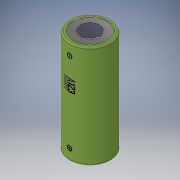
# Autodesk Inventor part: Battery Cell
Saved by Autodesk Inventor 2019.2 (Build 232265000, 265)
## iProperties
Created: 2018-12-05
Part Number: Battery Cell
Material: Nickel-Copper Alloy 400
Document SubType Name: Modeling
Designer: Petar
Density: 8.83 g/cm^3
Appearance: Chrome - Polished
Author: Petar
Autodesk Inventor part; units mm, degrees
ref_plane "YZ Plane" through (0, 0, 0) normal (1, 0, 0) x (0, 1, 0)
ref_plane "XZ Plane" through (0, 0, 0) normal (0, 1, 0) x (-1, 0, 0)
sketch "Sketch1" plane through (0, 0, 0) normal (1, 0, 0) x (0, 1, 0)
  line L0 (0, 0) -> (65, 0)
  line L1 (65, 0) -> (65, 13)
  line L2 (65, 13) -> (0, 13)
  line L3 (0, 13) -> (0, 0)
  dimension "d0" = 65
  dimension "d1" = 13
  constraints: 8 end point, 2 perpendicular, 1 horizontal, 1 vertical
  measures "d0" distance of L0.start L0.end
  measures "d1" distance of L0.end L1.end
revolve "Revolution1" add sketch "Sketch1" angle 360 about axis through (0, 0, 0) along (0, 1, 0)
fillet "Fillet1" radius 1 2 edges at (0, 65, -13) (0, 0, -13)
sketch "Sketch2" plane through (0, 65, 0) normal (0, 1, 0) x (1, 0, 0)
  circle A0 centre (0, 0) radius 12 projected
  circle A1 centre (0, 0) radius 6.5
  circle A2 centre (0, 0) radius 10.5
  dimension "d4" = 13
  dimension "d5" = 21
  constraints: 2 centre point, 2 coincident
  measures "d4" diameter of A1
  measures "d5" diameter of A2
extrude "Extrusion1" cut sketch "Sketch2" against normal blind 0.2 contours A2
fillet "Fillet2" radius 0.5 2 edges at (-10.5, 65, 0) (-6.5, 65, 0)
sketch "Sketch5" plane through (0, 0, 0) normal (0, -1, 0) x (1, 0, 0)
  circle A0 centre (0, 0) radius 10.9 projected
extrude "Extrusion2" cut sketch "Sketch5" against normal blind 0.2
ref_plane "Work Plane1" through (0, 65, 13) normal (0, 0, 1) x (1, 0, 0)
sketch "Sketch3" plane through (0, 65, 13) normal (0, 0, 1) x (1, 0, 0)
  line L0 (1.2249, -5) -> (1.2249, -9.446) construction
  line L1 (1.2249, -9.446) -> (-1.2249, -9.446) construction
  line L2 (-1.2249, -9.446) -> (-1.2249, -5) construction
  line L3 (-1.2249, -5) -> (1.2249, -5) construction
  line L4 (0, -65) -> (0, -0.9999) construction
  line L5 (1.8449, -55.554) -> (1.8449, -60) construction
  line L6 (1.8449, -60) -> (-1.8449, -60) construction
  line L7 (-1.8449, -60) -> (-1.8449, -55.554) construction
  line L8 (-1.8449, -55.554) -> (1.8449, -55.554) construction
  line L9 (-4.7875, -3) -> (4.7875, -3) construction
  line L10 (4.7875, -3) -> (4.7875, -11.446) construction
  line L11 (4.7875, -11.446) -> (-4.7875, -11.446) construction
  line L12 (-4.7875, -11.446) -> (-4.7875, -3) construction
  line L13 (-4.7783, -53.554) -> (4.7783, -53.554) construction
  line L14 (4.7783, -53.554) -> (4.7783, -62) construction
  line L15 (4.7783, -62) -> (-4.7783, -62) construction
  line L16 (-4.7783, -62) -> (-4.7783, -53.554) construction
  line L17 (13, -1) -> (-13, -1) construction
  line L18 (-13, -64) -> (13, -64) construction
  spline S0 degree 2 poles (1.1765, -6.0465) (1.3866, -6.2492) (1.6165, -6.8424) (1.6165, -7.223) knots 0 0 0 1 2 2 2
  spline S1 degree 2 poles (1.6165, -7.223) (1.6165, -7.5937) (1.3915, -8.1943) (1.1765, -8.397) knots 0 0 0 1 2 2 2
  spline S2 degree 2 poles (1.1765, -8.397) (0.9541, -8.6096) (0.3584, -8.8123) (0, -8.8123) knots 0 0 0 1 2 2 2
  spline S3 degree 2 poles (0, -8.8123) (-0.3707, -8.8123) (-0.9664, -8.6022) (-1.179, -8.397) knots 0 0 0 1 2 2 2
  spline S4 degree 2 poles (-1.179, -8.397) (-1.3915, -8.1943) (-1.6165, -7.5987) (-1.6165, -7.223) knots 0 0 0 1 2 2 2
  spline S5 degree 2 poles (-1.6165, -7.223) (-1.6165, -6.8399) (-1.3891, -6.2566) (-1.1765, -6.0465) knots 0 0 0 1 2 2 2
  spline S6 degree 2 poles (-1.1765, -6.0465) (-0.9664, -5.8438) (-0.3683, -5.6337) (0, -5.6337) knots 0 0 0 1 2 2 2
  spline S7 degree 2 poles (0, -5.6337) (0.3707, -5.6337) (0.9714, -5.8512) (1.1765, -6.0465) knots 0 0 0 1 2 2 2
  spline S8 degree 2 poles (1.1098, -7.223) (1.1098, -6.9214) (0.9541, -6.4543) (0.8107, -6.3011) knots 0 0 0 1 2 2 2
  spline S9 degree 2 poles (0.8107, -6.3011) (0.6649, -6.1429) (0.2571, -5.9847) (0.0025, -5.9847) knots 0 0 0 1 2 2 2
  spline S10 degree 2 poles (0.0025, -5.9847) (-0.2645, -5.9847) (-0.6575, -6.1379) (-0.8107, -6.3011) knots 0 0 0 1 2 2 2
  spline S11 degree 2 poles (-0.8107, -6.3011) (-0.9541, -6.4568) (-1.1098, -6.9264) (-1.1098, -7.223) knots 0 0 0 1 2 2 2
  spline S12 degree 2 poles (-1.1098, -7.223) (-1.1098, -7.8236) (-0.5067, -8.4613) (0.0025, -8.4613) knots 0 0 0 1 2 2 2
  spline S13 degree 2 poles (0.0025, -8.4613) (0.5092, -8.4613) (1.1098, -7.8236) (1.1098, -7.223) knots 0 0 0 1 2 2 2
  line L19 (-0.1957, -6.3278) -> (0.1957, -6.3278)
  line L20 (0.1957, -6.3278) -> (0.1957, -8.1206)
  line L21 (0.1957, -8.1206) -> (-0.1957, -8.1206)
  line L22 (-0.1957, -8.1206) -> (-0.1957, -6.3278)
  spline S14 degree 2 poles (1.1765, -56.6005) (1.3866, -56.8032) (1.6165, -57.3964) (1.6165, -57.777) knots 0 0 0 1 2 2 2
  spline S15 degree 2 poles (1.6165, -57.777) (1.6165, -58.1478) (1.3915, -58.7484) (1.1765, -58.951) knots 0 0 0 1 2 2 2
  spline S16 degree 2 poles (1.1765, -58.951) (0.9541, -59.1636) (0.3584, -59.3663) (0, -59.3663) knots 0 0 0 1 2 2 2
  spline S17 degree 2 poles (0, -59.3663) (-0.3707, -59.3663) (-0.9664, -59.1562) (-1.179, -58.951) knots 0 0 0 1 2 2 2
  spline S18 degree 2 poles (-1.179, -58.951) (-1.3915, -58.7484) (-1.6165, -58.1527) (-1.6165, -57.777) knots 0 0 0 1 2 2 2
  spline S19 degree 2 poles (-1.6165, -57.777) (-1.6165, -57.3939) (-1.3891, -56.8106) (-1.1765, -56.6005) knots 0 0 0 1 2 2 2
  spline S20 degree 2 poles (-1.1765, -56.6005) (-0.9664, -56.3978) (-0.3683, -56.1877) (0, -56.1877) knots 0 0 0 1 2 2 2
  spline S21 degree 2 poles (0, -56.1877) (0.3707, -56.1877) (0.9714, -56.4053) (1.1765, -56.6005) knots 0 0 0 1 2 2 2
  spline S22 degree 2 poles (1.1098, -57.777) (1.1098, -57.4755) (0.9541, -57.0083) (0.8107, -56.8551) knots 0 0 0 1 2 2 2
  spline S23 degree 2 poles (0.8107, -56.8551) (0.6649, -56.6969) (0.2571, -56.5387) (0.0025, -56.5387) knots 0 0 0 1 2 2 2
  spline S24 degree 2 poles (0.0025, -56.5387) (-0.2645, -56.5387) (-0.6575, -56.692) (-0.8107, -56.8551) knots 0 0 0 1 2 2 2
  spline S25 degree 2 poles (-0.8107, -56.8551) (-0.9541, -57.0108) (-1.1098, -57.4804) (-1.1098, -57.777) knots 0 0 0 1 2 2 2
  spline S26 degree 2 poles (-1.1098, -57.777) (-1.1098, -58.3776) (-0.5067, -59.0153) (0.0025, -59.0153) knots 0 0 0 1 2 2 2
  spline S27 degree 2 poles (0.0025, -59.0153) (0.5092, -59.0153) (1.1098, -58.3776) (1.1098, -57.777) knots 0 0 0 1 2 2 2
  line L23 (-1.0474, -57.5934) -> (-0.1776, -57.5934)
  line L24 (-0.1776, -57.5934) -> (-0.1776, -56.7308)
  line L25 (-0.1776, -56.7308) -> (0.1848, -56.7308)
  line L26 (0.1848, -56.7308) -> (0.1848, -57.5934)
  line L27 (0.1848, -57.5934) -> (1.0474, -57.5934)
  line L28 (1.0474, -57.5934) -> (1.0474, -57.9606)
  line L29 (1.0474, -57.9606) -> (0.1848, -57.9606)
  line L30 (0.1848, -57.9606) -> (0.1848, -58.8232)
  line L31 (0.1848, -58.8232) -> (-0.1776, -58.8232)
  line L32 (-0.1776, -58.8232) -> (-0.1776, -57.9606)
  line L33 (-0.1776, -57.9606) -> (-1.0474, -57.9606)
  line L34 (-1.0474, -57.9606) -> (-1.0474, -57.5934)
  dimension "d9" = 2
  dimension "d10" = 2
  dimension "d11" = 2
  dimension "d12" = 2
  dimension "d13" = 2
  dimension "d14" = 2
  constraints: 2 end point, 1 vertical, 12 other
  measures "d9" distance between parallel lines of L11 L1
  measures "d10" distance between parallel lines of L9 L3
  measures "d11" distance between parallel lines of L8 L13
  measures "d12" distance between parallel lines of L15 L6
  measures "d13" distance between parallel lines of L9 L17
  measures "d14" distance between parallel lines of L18 L15
emboss "Emboss1" sketch "Sketch3" operation cut depth 0.01 direction (0, 0, -1) draft 1
sketch "Sketch4" plane through (0, 65, 13) normal (0, 0, 1) x (1, 0, 0)
  line L0 (-6.1, 0) -> (6.1, 0) construction
  line L1 (0, 0) -> (0, -65) construction
  line L2 (3.5, -19) -> (3.5, -28) construction
  line L3 (3.5, -28) -> (-0.8355, -28) construction
  line L4 (-0.8355, -28) -> (-0.8355, -19) construction
  line L5 (-0.8355, -19) -> (3.5, -19) construction
  line L6 (-0.9355, -19) -> (-0.9355, -28) construction
  line L7 (-0.9355, -28) -> (-4.5, -28) construction
  line L8 (-4.5, -28) -> (-4.5, -19) construction
  line L9 (-4.5, -19) -> (-0.9355, -19) construction
  line L10 (3.2329, -20.5357) -> (-0.7671, -21.3601)
  line L11 (-0.7671, -21.3601) -> (-0.7671, -20.7321)
  line L12 (-0.7671, -20.7321) -> (-0.2046, -20.625)
  line L13 (-0.2046, -20.625) -> (-0.2046, -19.8363)
  line L14 (-0.2046, -19.8363) -> (-0.7671, -19.7351)
  line L15 (-0.7671, -19.7351) -> (-0.7671, -19.1071)
  line L16 (-0.7671, -19.1071) -> (3.2329, -19.9077)
  line L17 (3.2329, -19.9077) -> (3.2329, -20.5357)
  line L18 (0.2805, -19.9196) -> (0.2805, -20.5446)
  line L19 (0.2805, -20.5446) -> (2.1317, -20.2262)
  line L20 (2.1317, -20.2262) -> (0.2805, -19.9196)
  spline S0 degree 2 poles (2.9085, -21.7827) (2.9085, -21.9048) (3.0484, -22.006) (3.2329, -22.006) knots 0 0 0 1 2 2 2
  line L21 (3.2329, -22.006) -> (3.2329, -22.6607)
  line L22 (3.2329, -22.6607) -> (-0.7671, -22.6607)
  line L23 (-0.7671, -22.6607) -> (-0.7671, -22.006)
  line L24 (-0.7671, -22.006) -> (2.4234, -22.006)
  line L25 (2.4234, -22.006) -> (2.4234, -21.503)
  line L26 (2.4234, -21.503) -> (2.9085, -21.503)
  line L27 (2.9085, -21.503) -> (2.9085, -21.7827)
  spline S1 degree 2 poles (3.3014, -24.0208) (3.3014, -24.4583) (2.8668, -25.003) (2.3906, -25.003) knots 0 0 0 1 2 2 2
  spline S2 degree 2 poles (2.3906, -25.003) (2.1734, -25.003) (1.8639, -24.8839) (1.7002, -24.7738) knots 0 0 0 1 2 2 2
  spline S3 degree 2 poles (1.7002, -24.7738) (1.599, -24.7024) (1.3103, -24.4554) (1.0305, -24.2083) (0.7865, -24.0327) (0.6406, -23.9107) knots 0 0 0 1 2 3 4 4 4
  spline S4 degree 2 poles (0.6406, -23.9107) (0.5811, -23.878) (0.4353, -23.7946) (0.3073, -23.75) (0.1615, -23.7321) (0.0514, -23.7321) knots 0 0 0 1 2 3 4 4 4
  line L28 (0.0514, -23.7321) -> (-0.2225, -23.7321)
  line L29 (-0.2225, -23.7321) -> (-0.2225, -25.003)
  line L30 (-0.2225, -25.003) -> (-0.7671, -25.003)
  line L31 (-0.7671, -25.003) -> (-0.7671, -23.0774)
  line L32 (-0.7671, -23.0774) -> (0.0514, -23.0774)
  spline S5 degree 2 poles (0.0514, -23.0774) (0.2478, -23.0774) (0.6347, -23.1845) (0.8549, -23.3333) knots 0 0 0 1 2 2 2
  spline S6 degree 2 poles (0.8549, -23.3333) (0.9531, -23.4018) (1.227, -23.631) (1.5127, -23.875) (1.7805, -24.1071) (1.8906, -24.1815) knots 0 0 0 1 2 3 4 4 4
  spline S7 degree 2 poles (1.8906, -24.1815) (2.0335, -24.2798) (2.2805, -24.3542) (2.4055, -24.3542) knots 0 0 0 1 2 2 2
  spline S8 degree 2 poles (2.4055, -24.3542) (2.6049, -24.3542) (2.7567, -24.1786) (2.7567, -24.0089) knots 0 0 0 1 2 2 2
  spline S9 degree 2 poles (2.7567, -24.0089) (2.7567, -23.8304) (2.6168, -23.6488) (2.471, -23.6488) knots 0 0 0 1 2 2 2
  line L33 (2.471, -23.6488) -> (2.3014, -23.6488)
  line L34 (2.3014, -23.6488) -> (2.3014, -23.0357)
  line L35 (2.3014, -23.0357) -> (2.4799, -23.0357)
  spline S10 degree 2 poles (2.4799, -23.0357) (2.8609, -23.0357) (3.3014, -23.5536) (3.3014, -24.0208) knots 0 0 0 1 2 2 2
  spline S11 degree 2 poles (3.3014, -26.2411) (3.3014, -26.4851) (3.1674, -26.8542) (2.9264, -27.1131) (2.596, -27.2411) (2.4115, -27.2411) knots 0 0 0 1 2 3 4 4 4
  line L36 (2.4115, -27.2411) -> (1.8668, -27.2411)
  spline S12 degree 2 poles (1.8668, -27.2411) (1.6139, -27.2411) (1.3222, -27.0565) (1.3073, -26.8988) knots 0 0 0 1 2 2 2
  spline S13 degree 2 poles (1.3073, -26.8988) (1.2895, -27.0685) (0.9799, -27.2946) (0.7061, -27.2946) knots 0 0 0 1 2 2 2
  line L37 (0.7061, -27.2946) -> (-0.0201, -27.2946)
  spline S14 degree 2 poles (-0.0201, -27.2946) (-0.2105, -27.2946) (-0.5171, -27.1339) (-0.7284, -26.8542) (-0.8355, -26.4851) (-0.8355, -26.2708) knots 0 0 0 1 2 3 4 4 4
  spline S15 degree 2 poles (-0.8355, -26.2708) (-0.8355, -26.0565) (-0.7284, -25.6964) (-0.5111, -25.4286) (-0.2046, -25.2798) (-0.0141, -25.2798) knots 0 0 0 1 2 3 4 4 4
  line L38 (-0.0141, -25.2798) -> (0.2359, -25.2798)
  line L39 (0.2359, -25.2798) -> (0.1139, -25.8929)
  line L40 (0.1139, -25.8929) -> (-0.0052, -25.8929)
  spline S16 degree 2 poles (-0.0052, -25.8929) (-0.151, -25.8929) (-0.2939, -26.0893) (-0.2939, -26.2649) knots 0 0 0 1 2 2 2
  spline S17 degree 2 poles (-0.2939, -26.2649) (-0.2939, -26.4464) (-0.148, -26.6458) (-0.0052, -26.6458) knots 0 0 0 1 2 2 2
  line L41 (-0.0052, -26.6458) -> (0.7121, -26.6458)
  spline S18 degree 2 poles (0.7121, -26.6458) (0.8996, -26.6458) (1.0454, -26.4851) (1.0454, -26.2649) knots 0 0 0 1 2 2 2
  line L42 (1.0454, -26.2649) -> (1.0454, -25.8839)
  line L43 (1.0454, -25.8839) -> (1.5395, -25.8839)
  line L44 (1.5395, -25.8839) -> (1.5395, -26.2292)
  spline S19 degree 2 poles (1.5395, -26.2292) (1.5395, -26.4375) (1.6734, -26.5982) (1.852, -26.5982) knots 0 0 0 1 2 2 2
  line L45 (1.852, -26.5982) -> (2.4145, -26.5982)
  spline S20 degree 2 poles (2.4145, -26.5982) (2.5781, -26.5982) (2.7567, -26.4345) (2.7567, -26.2351) knots 0 0 0 1 2 2 2
  spline S21 degree 2 poles (2.7567, -26.2351) (2.7567, -26.0536) (2.6049, -25.8929) (2.4502, -25.8929) knots 0 0 0 1 2 2 2
  line L46 (2.4502, -25.8929) -> (2.3014, -25.8929)
  line L47 (2.3014, -25.8929) -> (2.3014, -25.2798)
  line L48 (2.3014, -25.2798) -> (2.4799, -25.2798)
  spline S22 degree 2 poles (2.4799, -25.2798) (2.8609, -25.2798) (3.3014, -25.8036) (3.3014, -26.2411) knots 0 0 0 1 2 2 2
  line L49 (-1.7706, -19.075) -> (-1.7578, -19.225)
  spline S23 degree 2 poles (-1.7578, -19.225) (-1.8484, -19.236) (-1.9636, -19.3137) (-2.0349, -19.4774) (-2.0349, -19.5799) knots 0 0 0 1 2 3 3 3
  spline S24 degree 2 poles (-2.0349, -19.5799) (-2.0349, -19.6704) (-1.981, -19.8104) (-1.8868, -19.878) (-1.831, -19.878) knots 0 0 0 1 2 3 3 3
  spline S25 degree 2 poles (-1.831, -19.878) (-1.7743, -19.878) (-1.6901, -19.8131) (-1.6618, -19.7372) knots 0 0 0 1 2 2 2
  spline S26 degree 2 poles (-1.6618, -19.7372) (-1.6426, -19.6887) (-1.563, -19.3567) (-1.5273, -19.2899) knots 0 0 0 1 2 2 2
  spline S27 degree 2 poles (-1.5273, -19.2899) (-1.4825, -19.204) (-1.349, -19.1198) (-1.2666, -19.1198) knots 0 0 0 1 2 2 2
  spline S28 degree 2 poles (-1.2666, -19.1198) (-1.1752, -19.1198) (-1.0179, -19.2232) (-0.9355, -19.4216) (-0.9355, -19.5433) knots 0 0 0 1 2 3 3 3
  spline S29 degree 2 poles (-0.9355, -19.5433) (-0.9355, -19.6768) (-1.0215, -19.8808) (-1.1889, -19.9915) (-1.2941, -19.9951) knots 0 0 0 1 2 3 3 3
  line L50 (-1.2941, -19.9951) -> (-1.306, -19.8433)
  spline S30 degree 2 poles (-1.306, -19.8433) (-1.1916, -19.8314) (-1.0755, -19.6887) (-1.0755, -19.5497) knots 0 0 0 1 2 2 2
  spline S31 degree 2 poles (-1.0755, -19.5497) (-1.0755, -19.4052) (-1.1816, -19.2726) (-1.2557, -19.2726) knots 0 0 0 1 2 2 2
  spline S32 degree 2 poles (-1.2557, -19.2726) (-1.3206, -19.2726) (-1.3627, -19.3192) knots 0 0 0 1 1 1
  spline S33 degree 2 poles (-1.3627, -19.3192) (-1.4038, -19.3659) (-1.4916, -19.7546) (-1.5246, -19.8268) knots 0 0 0 1 2 2 2
  spline S34 degree 2 poles (-1.5246, -19.8268) (-1.573, -19.9311) (-1.7212, -20.0308) (-1.8173, -20.0308) knots 0 0 0 1 2 2 2
  spline S35 degree 2 poles (-1.8173, -20.0308) (-1.9133, -20.0308) (-2.0825, -19.921) (-2.1767, -19.7152) (-2.1767, -19.5872) knots 0 0 0 1 2 3 3 3
  spline S36 degree 2 poles (-2.1767, -19.5872) (-2.1767, -19.4235) (-2.0816, -19.204) (-1.8913, -19.0787) (-1.7706, -19.075) knots 0 0 0 1 2 3 3 3
  line L51 (-2.1566, -20.586) -> (-1.648, -20.586)
  line L52 (-1.648, -20.586) -> (-0.9566, -20.1232)
  line L53 (-0.9566, -20.1232) -> (-0.9566, -20.3162)
  line L54 (-0.9566, -20.3162) -> (-1.3188, -20.553)
  spline S37 degree 2 poles (-1.3188, -20.553) (-1.4194, -20.6198) (-1.5218, -20.6756) knots 0 0 0 1 1 1
  spline S38 degree 2 poles (-1.5218, -20.6756) (-1.4276, -20.7296) (-1.3096, -20.8064) knots 0 0 0 1 1 1
  line L55 (-1.3096, -20.8064) -> (-0.9566, -21.0396)
  line L56 (-0.9566, -21.0396) -> (-0.9566, -21.2244)
  line L57 (-0.9566, -21.2244) -> (-1.648, -20.7451)
  line L58 (-1.648, -20.7451) -> (-2.1566, -20.7451)
  line L59 (-2.1566, -20.7451) -> (-2.1566, -20.586)
  line L60 (-1.7706, -21.3122) -> (-1.7578, -21.4622)
  spline S39 degree 2 poles (-1.7578, -21.4622) (-1.8484, -21.4732) (-1.9636, -21.5509) (-2.0349, -21.7146) (-2.0349, -21.8171) knots 0 0 0 1 2 3 3 3
  spline S40 degree 2 poles (-2.0349, -21.8171) (-2.0349, -21.9076) (-1.981, -22.0476) (-1.8868, -22.1152) (-1.831, -22.1152) knots 0 0 0 1 2 3 3 3
  spline S41 degree 2 poles (-1.831, -22.1152) (-1.7743, -22.1152) (-1.6901, -22.0503) (-1.6618, -21.9744) knots 0 0 0 1 2 2 2
  spline S42 degree 2 poles (-1.6618, -21.9744) (-1.6426, -21.9259) (-1.563, -21.5939) (-1.5273, -21.5271) knots 0 0 0 1 2 2 2
  spline S43 degree 2 poles (-1.5273, -21.5271) (-1.4825, -21.4412) (-1.349, -21.357) (-1.2666, -21.357) knots 0 0 0 1 2 2 2
  spline S44 degree 2 poles (-1.2666, -21.357) (-1.1752, -21.357) (-1.0179, -21.4604) (-0.9355, -21.6588) (-0.9355, -21.7805) knots 0 0 0 1 2 3 3 3
  spline S45 degree 2 poles (-0.9355, -21.7805) (-0.9355, -21.914) (-1.0215, -22.118) (-1.1889, -22.2287) (-1.2941, -22.2323) knots 0 0 0 1 2 3 3 3
  line L61 (-1.2941, -22.2323) -> (-1.306, -22.0805)
  spline S46 degree 2 poles (-1.306, -22.0805) (-1.1916, -22.0686) (-1.0755, -21.9259) (-1.0755, -21.7869) knots 0 0 0 1 2 2 2
  spline S47 degree 2 poles (-1.0755, -21.7869) (-1.0755, -21.6424) (-1.1816, -21.5098) (-1.2557, -21.5098) knots 0 0 0 1 2 2 2
  spline S48 degree 2 poles (-1.2557, -21.5098) (-1.3206, -21.5098) (-1.3627, -21.5564) knots 0 0 0 1 1 1
  spline S49 degree 2 poles (-1.3627, -21.5564) (-1.4038, -21.603) (-1.4916, -21.9918) (-1.5246, -22.064) knots 0 0 0 1 2 2 2
  spline S50 degree 2 poles (-1.5246, -22.064) (-1.573, -22.1683) (-1.7212, -22.268) (-1.8173, -22.268) knots 0 0 0 1 2 2 2
  spline S51 degree 2 poles (-1.8173, -22.268) (-1.9133, -22.268) (-2.0825, -22.1582) (-2.1767, -21.9524) (-2.1767, -21.8244) knots 0 0 0 1 2 3 3 3
  spline S52 degree 2 poles (-2.1767, -21.8244) (-2.1767, -21.6607) (-2.0816, -21.4412) (-1.8913, -21.3159) (-1.7706, -21.3122) knots 0 0 0 1 2 3 3 3
  line L62 (-2.1566, -22.7902) -> (-1.0984, -22.7902)
  line L63 (-1.0984, -22.7902) -> (-1.0984, -22.3951)
  line L64 (-1.0984, -22.3951) -> (-0.9566, -22.3951)
  line L65 (-0.9566, -22.3951) -> (-0.9566, -23.3463)
  line L66 (-0.9566, -23.3463) -> (-1.0984, -23.3463)
  line L67 (-1.0984, -23.3463) -> (-1.0984, -22.9494)
  line L68 (-1.0984, -22.9494) -> (-2.1566, -22.9494)
  line L69 (-2.1566, -22.9494) -> (-2.1566, -22.7902)
  line L70 (-2.1566, -23.5128) -> (-0.9566, -23.5128)
  line L71 (-0.9566, -23.5128) -> (-0.9566, -24.3817)
  line L72 (-0.9566, -24.3817) -> (-1.0984, -24.3817)
  line L73 (-1.0984, -24.3817) -> (-1.0984, -23.672)
  line L74 (-1.0984, -23.672) -> (-1.4651, -23.672)
  line L75 (-1.4651, -23.672) -> (-1.4651, -24.3369)
  line L76 (-1.4651, -24.3369) -> (-1.6069, -24.3369)
  line L77 (-1.6069, -24.3369) -> (-1.6069, -23.672)
  line L78 (-1.6069, -23.672) -> (-2.0148, -23.672)
  line L79 (-2.0148, -23.672) -> (-2.0148, -24.4091)
  line L80 (-2.0148, -24.4091) -> (-2.1566, -24.4091)
  line L81 (-2.1566, -24.4091) -> (-2.1566, -23.5128)
  line L82 (-2.1566, -24.6232) -> (-0.9566, -24.6232)
  line L83 (-0.9566, -24.6232) -> (-0.9566, -24.8619)
  line L84 (-0.9566, -24.8619) -> (-1.8063, -25.1463)
  spline S53 degree 2 poles (-1.8063, -25.1463) (-1.9252, -25.1857) (-1.9837, -25.204) knots 0 0 0 1 1 1
  spline S54 degree 2 poles (-1.9837, -25.204) (-1.9188, -25.2241) (-1.7916, -25.268) knots 0 0 0 1 1 1
  line L85 (-1.7916, -25.268) -> (-0.9566, -25.5561)
  line L86 (-0.9566, -25.5561) -> (-0.9566, -25.7692)
  line L87 (-0.9566, -25.7692) -> (-2.1566, -25.7692)
  line L88 (-2.1566, -25.7692) -> (-2.1566, -25.6165)
  line L89 (-2.1566, -25.6165) -> (-1.1523, -25.6165)
  line L90 (-1.1523, -25.6165) -> (-2.1566, -25.2662)
  line L91 (-2.1566, -25.2662) -> (-2.1566, -25.1235)
  line L92 (-2.1566, -25.1235) -> (-1.1349, -24.7759)
  line L93 (-1.1349, -24.7759) -> (-2.1566, -24.7759)
  line L94 (-2.1566, -24.7759) -> (-2.1566, -24.6232)
  line L95 (-1.7706, -25.9704) -> (-1.7578, -26.1204)
  spline S55 degree 2 poles (-1.7578, -26.1204) (-1.8484, -26.1314) (-1.9636, -26.2091) (-2.0349, -26.3729) (-2.0349, -26.4753) knots 0 0 0 1 2 3 3 3
  spline S56 degree 2 poles (-2.0349, -26.4753) (-2.0349, -26.5659) (-1.981, -26.7058) (-1.8868, -26.7735) (-1.831, -26.7735) knots 0 0 0 1 2 3 3 3
  spline S57 degree 2 poles (-1.831, -26.7735) (-1.7743, -26.7735) (-1.6901, -26.7085) (-1.6618, -26.6326) knots 0 0 0 1 2 2 2
  spline S58 degree 2 poles (-1.6618, -26.6326) (-1.6426, -26.5841) (-1.563, -26.2521) (-1.5273, -26.1854) knots 0 0 0 1 2 2 2
  spline S59 degree 2 poles (-1.5273, -26.1854) (-1.4825, -26.0994) (-1.349, -26.0152) (-1.2666, -26.0152) knots 0 0 0 1 2 2 2
  spline S60 degree 2 poles (-1.2666, -26.0152) (-1.1752, -26.0152) (-1.0179, -26.1186) (-0.9355, -26.3171) (-0.9355, -26.4387) knots 0 0 0 1 2 3 3 3
  spline S61 degree 2 poles (-0.9355, -26.4387) (-0.9355, -26.5723) (-1.0215, -26.7762) (-1.1889, -26.8869) (-1.2941, -26.8905) knots 0 0 0 1 2 3 3 3
  line L96 (-1.2941, -26.8905) -> (-1.306, -26.7387)
  spline S62 degree 2 poles (-1.306, -26.7387) (-1.1916, -26.7268) (-1.0755, -26.5841) (-1.0755, -26.4451) knots 0 0 0 1 2 2 2
  spline S63 degree 2 poles (-1.0755, -26.4451) (-1.0755, -26.3006) (-1.1816, -26.168) (-1.2557, -26.168) knots 0 0 0 1 2 2 2
  spline S64 degree 2 poles (-1.2557, -26.168) (-1.3206, -26.168) (-1.3627, -26.2146) knots 0 0 0 1 1 1
  spline S65 degree 2 poles (-1.3627, -26.2146) (-1.4038, -26.2613) (-1.4916, -26.65) (-1.5246, -26.7223) knots 0 0 0 1 2 2 2
  spline S66 degree 2 poles (-1.5246, -26.7223) (-1.573, -26.8265) (-1.7212, -26.9262) (-1.8173, -26.9262) knots 0 0 0 1 2 2 2
  spline S67 degree 2 poles (-1.8173, -26.9262) (-1.9133, -26.9262) (-2.0825, -26.8165) (-2.1767, -26.6107) (-2.1767, -26.4826) knots 0 0 0 1 2 3 3 3
  spline S68 degree 2 poles (-2.1767, -26.4826) (-2.1767, -26.3189) (-2.0816, -26.0994) (-1.8913, -25.9741) (-1.7706, -25.9704) knots 0 0 0 1 2 3 3 3
  line L97 (-3.5689, -18.9988) -> (-2.7689, -19.3061)
  line L98 (-2.7689, -19.3061) -> (-2.7689, -19.4207)
  line L99 (-2.7689, -19.4207) -> (-3.5689, -19.7476)
  line L100 (-3.5689, -19.7476) -> (-3.5689, -19.6268)
  line L101 (-3.5689, -19.6268) -> (-3.3268, -19.5341)
  line L102 (-3.3268, -19.5341) -> (-3.3268, -19.1988)
  line L103 (-3.3268, -19.1988) -> (-3.5689, -19.111)
  line L104 (-3.5689, -19.111) -> (-3.5689, -18.9988)
  line L105 (-3.2409, -19.2293) -> (-3.2409, -19.5012)
  line L106 (-3.2409, -19.5012) -> (-3.0189, -19.4171)
  spline S69 degree 2 poles (-3.0189, -19.4171) (-2.9177, -19.3793) (-2.8531, -19.361) knots 0 0 0 1 1 1
  spline S70 degree 2 poles (-2.8531, -19.361) (-2.9299, -19.3451) (-3.0061, -19.3177) knots 0 0 0 1 1 1
  line L107 (-3.0061, -19.3177) -> (-3.2409, -19.2293)
  line L108 (-3.5689, -19.8311) -> (-2.7689, -19.8311)
  line L109 (-2.7689, -19.8311) -> (-2.7689, -19.9396)
  line L110 (-2.7689, -19.9396) -> (-3.397, -20.3604)
  line L111 (-3.397, -20.3604) -> (-2.7689, -20.3604)
  line L112 (-2.7689, -20.3604) -> (-2.7689, -20.4616)
  line L113 (-2.7689, -20.4616) -> (-3.5689, -20.4616)
  line L114 (-3.5689, -20.4616) -> (-3.5689, -20.353)
  line L115 (-3.5689, -20.353) -> (-2.9409, -19.9323)
  line L116 (-2.9409, -19.9323) -> (-3.5689, -19.9323)
  line L117 (-3.5689, -19.9323) -> (-3.5689, -19.8311)
  line L118 (-3.5689, -20.6409) -> (-2.7689, -20.6409)
  line L119 (-2.7689, -20.6409) -> (-2.7689, -20.9957)
  spline S71 degree 2 poles (-2.7689, -20.9957) (-2.7689, -21.1024) (-2.8122, -21.214) (-2.9213, -21.2805) (-2.9872, -21.2805) knots 0 0 0 1 2 3 3 3
  spline S72 degree 2 poles (-2.9872, -21.2805) (-3.0726, -21.2805) (-3.189, -21.1701) (-3.2049, -21.0555) knots 0 0 0 1 2 2 2
  spline S73 degree 2 poles (-3.2049, -21.0555) (-3.225, -21.097) (-3.2445, -21.1189) knots 0 0 0 1 1 1
  spline S74 degree 2 poles (-3.2445, -21.1189) (-3.2872, -21.1652) (-3.3512, -21.2067) knots 0 0 0 1 1 1
  line L120 (-3.3512, -21.2067) -> (-3.5689, -21.3451)
  line L121 (-3.5689, -21.3451) -> (-3.5689, -21.2128)
  line L122 (-3.5689, -21.2128) -> (-3.4024, -21.1067)
  spline S75 degree 2 poles (-3.4024, -21.1067) (-3.3305, -21.0604) (-3.2543, -21.0006) (-3.2232, -20.953) (-3.2171, -20.9287) knots 0 0 0 1 2 3 3 3
  spline S76 degree 2 poles (-3.2171, -20.9287) (-3.2134, -20.9104) (-3.2134, -20.8695) knots 0 0 0 1 1 1
  line L123 (-3.2134, -20.8695) -> (-3.2134, -20.747)
  line L124 (-3.2134, -20.747) -> (-3.5689, -20.747)
  line L125 (-3.5689, -20.747) -> (-3.5689, -20.6409)
  line L126 (-3.122, -20.747) -> (-3.122, -20.9744)
  spline S77 degree 2 poles (-3.122, -20.9744) (-3.122, -21.047) (-3.0921, -21.1287) (-3.0256, -21.1713) (-2.9872, -21.1713) knots 0 0 0 1 2 3 3 3
  spline S78 degree 2 poles (-2.9872, -21.1713) (-2.9305, -21.1713) (-2.8573, -21.089) (-2.8573, -21) knots 0 0 0 1 2 2 2
  line L127 (-2.8573, -21) -> (-2.8573, -20.747)
  line L128 (-2.8573, -20.747) -> (-3.122, -20.747)
  line L129 (-3.4744, -21.9226) -> (-3.5689, -21.9226)
  line L130 (-3.5689, -21.9226) -> (-3.5689, -21.3939)
  spline S79 degree 2 poles (-3.5689, -21.3939) (-3.5335, -21.3927) (-3.5006, -21.4055) knots 0 0 0 1 1 1
  spline S80 degree 2 poles (-3.5006, -21.4055) (-3.4463, -21.4256) (-3.3421, -21.5146) (-3.2732, -21.5988) knots 0 0 0 1 2 2 2
  spline S81 degree 2 poles (-3.2732, -21.5988) (-3.1659, -21.7287) (-3.0415, -21.8201) (-2.9854, -21.8201) knots 0 0 0 1 2 2 2
  spline S82 degree 2 poles (-2.9854, -21.8201) (-2.9268, -21.8201) (-2.847, -21.7366) (-2.847, -21.6695) knots 0 0 0 1 2 2 2
  spline S83 degree 2 poles (-2.847, -21.6695) (-2.847, -21.5988) (-2.9323, -21.514) (-3.0073, -21.5134) knots 0 0 0 1 2 2 2
  line L131 (-3.0073, -21.5134) -> (-2.997, -21.4122)
  spline S84 degree 2 poles (-2.997, -21.4122) (-2.8841, -21.4226) (-2.7659, -21.5579) (-2.7659, -21.672) knots 0 0 0 1 2 2 2
  spline S85 degree 2 poles (-2.7659, -21.672) (-2.7659, -21.7872) (-2.8933, -21.9213) (-2.9878, -21.9213) knots 0 0 0 1 2 2 2
  spline S86 degree 2 poles (-2.9878, -21.9213) (-3.036, -21.9213) (-3.1287, -21.8823) (-3.2311, -21.7909) (-3.3207, -21.6854) knots 0 0 0 1 2 3 3 3
  spline S87 degree 2 poles (-3.3207, -21.6854) (-3.3945, -21.597) (-3.4476, -21.547) (-3.4744, -21.5305) knots 0 0 0 1 2 2 2
  line L132 (-3.4744, -21.5305) -> (-3.4744, -21.9226)
  line L133 (-2.9652, -22.5384) -> (-2.9732, -22.4409)
  spline S88 degree 2 poles (-2.9732, -22.4409) (-2.9152, -22.4274) (-2.8884, -22.4037) knots 0 0 0 1 1 1
  spline S89 degree 2 poles (-2.8884, -22.4037) (-2.8463, -22.3634) (-2.8463, -22.3049) knots 0 0 0 1 1 1
  spline S90 degree 2 poles (-2.8463, -22.3049) (-2.8463, -22.2579) (-2.8726, -22.2226) knots 0 0 0 1 1 1
  spline S91 degree 2 poles (-2.8726, -22.2226) (-2.9061, -22.1762) (-3.0366, -22.1226) (-3.1567, -22.1213) knots 0 0 0 1 2 2 2
  spline S92 degree 2 poles (-3.1567, -22.1213) (-3.1024, -22.1567) (-3.05, -22.2598) (-3.05, -22.3159) knots 0 0 0 1 2 2 2
  spline S93 degree 2 poles (-3.05, -22.3159) (-3.05, -22.414) (-3.1945, -22.5524) (-3.3091, -22.5524) knots 0 0 0 1 2 2 2
  spline S94 degree 2 poles (-3.3091, -22.5524) (-3.3841, -22.5524) (-3.5134, -22.4872) (-3.5823, -22.3738) (-3.5823, -22.3018) knots 0 0 0 1 2 3 3 3
  spline S95 degree 2 poles (-3.5823, -22.3018) (-3.5823, -22.1787) (-3.4018, -22.0238) (-3.1945, -22.0238) knots 0 0 0 1 2 2 2
  spline S96 degree 2 poles (-3.1945, -22.0238) (-2.9628, -22.0238) (-2.8573, -22.1098) knots 0 0 0 1 1 1
  spline S97 degree 2 poles (-2.8573, -22.1098) (-2.7659, -22.1841) (-2.7659, -22.311) knots 0 0 0 1 1 1
  spline S98 degree 2 poles (-2.7659, -22.311) (-2.7659, -22.4055) (-2.872, -22.5262) (-2.9652, -22.5384) knots 0 0 0 1 2 2 2
  spline S99 degree 2 poles (-3.3098, -22.1366) (-3.3604, -22.1366) (-3.4531, -22.1799) (-3.5018, -22.2567) (-3.5018, -22.2994) knots 0 0 0 1 2 3 3 3
  spline S100 degree 2 poles (-3.5018, -22.2994) (-3.5018, -22.3622) (-3.4012, -22.4512) (-3.3152, -22.4512) knots 0 0 0 1 2 2 2
  spline S101 degree 2 poles (-3.3152, -22.4512) (-3.2323, -22.4512) (-3.1366, -22.3634) (-3.1366, -22.2957) knots 0 0 0 1 2 2 2
  spline S102 degree 2 poles (-3.1366, -22.2957) (-3.1366, -22.2293) (-3.2323, -22.1366) (-3.3098, -22.1366) knots 0 0 0 1 2 2 2
  line L134 (-2.9652, -23.1598) -> (-2.9732, -23.0622)
  spline S103 degree 2 poles (-2.9732, -23.0622) (-2.9152, -23.0488) (-2.8884, -23.025) knots 0 0 0 1 1 1
  spline S104 degree 2 poles (-2.8884, -23.025) (-2.8463, -22.9848) (-2.8463, -22.9262) knots 0 0 0 1 1 1
  spline S105 degree 2 poles (-2.8463, -22.9262) (-2.8463, -22.8793) (-2.8726, -22.8439) knots 0 0 0 1 1 1
  spline S106 degree 2 poles (-2.8726, -22.8439) (-2.9061, -22.7976) (-3.0366, -22.7439) (-3.1567, -22.7427) knots 0 0 0 1 2 2 2
  spline S107 degree 2 poles (-3.1567, -22.7427) (-3.1024, -22.778) (-3.05, -22.8811) (-3.05, -22.9372) knots 0 0 0 1 2 2 2
  spline S108 degree 2 poles (-3.05, -22.9372) (-3.05, -23.0354) (-3.1945, -23.1738) (-3.3091, -23.1738) knots 0 0 0 1 2 2 2
  spline S109 degree 2 poles (-3.3091, -23.1738) (-3.3841, -23.1738) (-3.5134, -23.1085) (-3.5823, -22.9951) (-3.5823, -22.9232) knots 0 0 0 1 2 3 3 3
  spline S110 degree 2 poles (-3.5823, -22.9232) (-3.5823, -22.8) (-3.4018, -22.6451) (-3.1945, -22.6451) knots 0 0 0 1 2 2 2
  spline S111 degree 2 poles (-3.1945, -22.6451) (-2.9628, -22.6451) (-2.8573, -22.7311) knots 0 0 0 1 1 1
  spline S112 degree 2 poles (-2.8573, -22.7311) (-2.7659, -22.8055) (-2.7659, -22.9323) knots 0 0 0 1 1 1
  spline S113 degree 2 poles (-2.7659, -22.9323) (-2.7659, -23.0268) (-2.872, -23.1476) (-2.9652, -23.1598) knots 0 0 0 1 2 2 2
  spline S114 degree 2 poles (-3.3098, -22.7579) (-3.3604, -22.7579) (-3.4531, -22.8012) (-3.5018, -22.878) (-3.5018, -22.9207) knots 0 0 0 1 2 3 3 3
  spline S115 degree 2 poles (-3.5018, -22.9207) (-3.5018, -22.9835) (-3.4012, -23.0726) (-3.3152, -23.0726) knots 0 0 0 1 2 2 2
  spline S116 degree 2 poles (-3.3152, -23.0726) (-3.2323, -23.0726) (-3.1366, -22.9848) (-3.1366, -22.9171) knots 0 0 0 1 2 2 2
  spline S117 degree 2 poles (-3.1366, -22.9171) (-3.1366, -22.8506) (-3.2323, -22.7579) (-3.3098, -22.7579) knots 0 0 0 1 2 2 2
  line L135 (-3.3591, -23.2707) -> (-3.3506, -23.3738)
  spline S118 degree 2 poles (-3.3506, -23.3738) (-3.4262, -23.3854) (-3.5018, -23.4683) (-3.5018, -23.5274) knots 0 0 0 1 2 2 2
  spline S119 degree 2 poles (-3.5018, -23.5274) (-3.5018, -23.5994) (-3.3945, -23.697) (-3.3061, -23.697) knots 0 0 0 1 2 2 2
  spline S120 degree 2 poles (-3.3061, -23.697) (-3.222, -23.697) (-3.1244, -23.603) (-3.1244, -23.5262) knots 0 0 0 1 2 2 2
  spline S121 degree 2 poles (-3.1244, -23.5262) (-3.1244, -23.4787) (-3.1677, -23.4024) (-3.2024, -23.3805) knots 0 0 0 1 2 2 2
  line L136 (-3.2024, -23.3805) -> (-3.1902, -23.2884)
  line L137 (-3.1902, -23.2884) -> (-2.7793, -23.3659)
  line L138 (-2.7793, -23.3659) -> (-2.7793, -23.7634)
  line L139 (-2.7793, -23.7634) -> (-2.8732, -23.7634)
  line L140 (-2.8732, -23.7634) -> (-2.8732, -23.4445)
  line L141 (-2.8732, -23.4445) -> (-3.0878, -23.4012)
  spline S122 degree 2 poles (-3.0878, -23.4012) (-3.0378, -23.4732) (-3.0378, -23.5524) knots 0 0 0 1 1 1
  spline S123 degree 2 poles (-3.0378, -23.5524) (-3.0378, -23.6573) (-3.1829, -23.8012) (-3.297, -23.8012) knots 0 0 0 1 2 2 2
  spline S124 degree 2 poles (-3.297, -23.8012) (-3.4061, -23.8012) (-3.4854, -23.7378) knots 0 0 0 1 1 1
  spline S125 degree 2 poles (-3.4854, -23.7378) (-3.5823, -23.661) (-3.5823, -23.528) knots 0 0 0 1 1 1
  spline S126 degree 2 poles (-3.5823, -23.528) (-3.5823, -23.4189) (-3.4604, -23.2805) (-3.3591, -23.2707) knots 0 0 0 1 2 2 2
  spline S127 degree 2 poles (-3.1744, -23.8921) (-3.0323, -23.8921) (-2.8591, -23.9506) (-2.7659, -24.0652) (-2.7659, -24.153) knots 0 0 0 1 2 3 3 3
  spline S128 degree 2 poles (-2.7659, -24.153) (-2.7659, -24.2171) (-2.8177, -24.3146) (-2.9152, -24.3774) (-3.0555, -24.4134) (-3.1744, -24.4134) knots 0 0 0 1 2 3 4 4 4
  spline S129 degree 2 poles (-3.1744, -24.4134) (-3.3152, -24.4134) (-3.4884, -24.3555) (-3.5823, -24.2402) (-3.5823, -24.153) knots 0 0 0 1 2 3 3 3
  spline S130 degree 2 poles (-3.5823, -24.153) (-3.5823, -24.0372) (-3.5, -23.9713) knots 0 0 0 1 1 1
  spline S131 degree 2 poles (-3.5, -23.9713) (-3.3994, -23.8921) (-3.1744, -23.8921) knots 0 0 0 1 1 1
  spline S132 degree 2 poles (-3.1744, -23.9933) (-3.372, -23.9933) (-3.5018, -24.0854) (-3.5018, -24.153) knots 0 0 0 1 2 2 2
  spline S133 degree 2 poles (-3.5018, -24.153) (-3.5018, -24.2201) (-3.3713, -24.3122) (-3.1744, -24.3122) knots 0 0 0 1 2 2 2
  spline S134 degree 2 poles (-3.1744, -24.3122) (-2.9768, -24.3122) (-2.847, -24.2201) (-2.847, -24.1518) knots 0 0 0 1 2 2 2
  spline S135 degree 2 poles (-2.847, -24.1518) (-2.847, -24.0841) (-2.9043, -24.0439) knots 0 0 0 1 1 1
  spline S136 degree 2 poles (-2.9043, -24.0439) (-2.9774, -23.9933) (-3.1744, -23.9933) knots 0 0 0 1 1 1
  line L142 (-3.5689, -24.5409) -> (-2.989, -24.5409)
  line L143 (-2.989, -24.5409) -> (-2.989, -24.6287)
  line L144 (-2.989, -24.6287) -> (-3.0707, -24.6287)
  spline S137 degree 2 poles (-3.0707, -24.6287) (-3.0281, -24.6561) (-2.9762, -24.7463) (-2.9762, -24.8043) knots 0 0 0 1 2 2 2
  spline S138 degree 2 poles (-2.9762, -24.8043) (-2.9762, -24.8689) (-3.0299, -24.9512) (-3.0781, -24.9683) knots 0 0 0 1 2 2 2
  spline S139 degree 2 poles (-3.0781, -24.9683) (-2.9762, -25.0372) (-2.9762, -25.1476) knots 0 0 0 1 1 1
  spline S140 degree 2 poles (-2.9762, -25.1476) (-2.9762, -25.2335) (-3.072, -25.3268) (-3.1713, -25.3268) knots 0 0 0 1 2 2 2
  line L145 (-3.1713, -25.3268) -> (-3.5689, -25.3268)
  line L146 (-3.5689, -25.3268) -> (-3.5689, -25.2287)
  line L147 (-3.5689, -25.2287) -> (-3.2037, -25.2287)
  spline S141 degree 2 poles (-3.2037, -25.2287) (-3.1451, -25.2287) (-3.0933, -25.2091) (-3.0616, -25.1591) (-3.0616, -25.1256) knots 0 0 0 1 2 3 3 3
  spline S142 degree 2 poles (-3.0616, -25.1256) (-3.0616, -25.064) (-3.1427, -24.9835) (-3.2323, -24.9835) knots 0 0 0 1 2 2 2
  line L148 (-3.2323, -24.9835) -> (-3.5689, -24.9835)
  line L149 (-3.5689, -24.9835) -> (-3.5689, -24.8854)
  line L150 (-3.5689, -24.8854) -> (-3.1927, -24.8854)
  spline S143 degree 2 poles (-3.1927, -24.8854) (-3.1268, -24.8854) (-3.0616, -24.8372) (-3.0616, -24.7823) knots 0 0 0 1 2 2 2
  spline S144 degree 2 poles (-3.0616, -24.7823) (-3.0616, -24.7409) (-3.1055, -24.6707) (-3.189, -24.639) (-3.2683, -24.639) knots 0 0 0 1 2 3 3 3
  line L151 (-3.2683, -24.639) -> (-3.5689, -24.639)
  line L152 (-3.5689, -24.639) -> (-3.5689, -24.5409)
  line L153 (-3.5689, -25.814) -> (-3.5689, -25.7159)
  line L154 (-3.5689, -25.7159) -> (-2.9433, -25.7159)
  spline S145 degree 2 poles (-2.9433, -25.7159) (-2.9768, -25.6805) (-3.0445, -25.5652) (-3.0616, -25.5195) knots 0 0 0 1 2 2 2
  line L155 (-3.0616, -25.5195) -> (-2.9665, -25.5195)
  spline S146 degree 2 poles (-2.9665, -25.5195) (-2.9281, -25.6018) (-2.8177, -25.725) (-2.7659, -25.7506) knots 0 0 0 1 2 2 2
  line L156 (-2.7659, -25.7506) -> (-2.7659, -25.814)
  line L157 (-2.7659, -25.814) -> (-3.5689, -25.814)
  line L158 (-3.5689, -26.1012) -> (-2.7689, -26.1012)
  line L159 (-2.7689, -26.1012) -> (-2.7689, -26.4012)
  spline S147 degree 2 poles (-2.7689, -26.4012) (-2.7689, -26.4927) (-2.8177, -26.6037) (-2.9183, -26.6665) (-2.9738, -26.6665) knots 0 0 0 1 2 3 3 3
  spline S148 degree 2 poles (-2.9738, -26.6665) (-3.025, -26.6665) (-3.1152, -26.611) (-3.1433, -26.5543) knots 0 0 0 1 2 2 2
  spline S149 degree 2 poles (-3.1433, -26.5543) (-3.1646, -26.6274) (-3.2671, -26.7055) (-3.3372, -26.7055) knots 0 0 0 1 2 2 2
  spline S150 degree 2 poles (-3.3372, -26.7055) (-3.3933, -26.7055) (-3.4896, -26.6579) (-3.5421, -26.5884) (-3.5689, -26.4829) (-3.5689, -26.4061) knots 0 0 0 1 2 3 4 4 4
  line L160 (-3.5689, -26.4061) -> (-3.5689, -26.1012)
  line L161 (-3.4744, -26.2073) -> (-3.4744, -26.4067)
  spline S151 degree 2 poles (-3.4744, -26.4067) (-3.4744, -26.4579) (-3.4707, -26.4787) knots 0 0 0 1 1 1
  spline S152 degree 2 poles (-3.4707, -26.4787) (-3.464, -26.5152) (-3.4335, -26.5646) (-3.375, -26.5963) (-3.3366, -26.5963) knots 0 0 0 1 2 3 3 3
  spline S153 degree 2 poles (-3.3366, -26.5963) (-3.2921, -26.5963) (-3.2262, -26.5494) (-3.1994, -26.4683) (-3.1994, -26.3921) knots 0 0 0 1 2 3 3 3
  line L162 (-3.1994, -26.3921) -> (-3.1994, -26.2073)
  line L163 (-3.1994, -26.2073) -> (-3.4744, -26.2073)
  line L164 (-3.1049, -26.2073) -> (-3.1049, -26.3799)
  spline S154 degree 2 poles (-3.1049, -26.3799) (-3.1049, -26.4506) (-3.0957, -26.4811) knots 0 0 0 1 1 1
  spline S155 degree 2 poles (-3.0957, -26.4811) (-3.0835, -26.5213) (-3.0281, -26.5622) (-2.986, -26.5622) knots 0 0 0 1 2 2 2
  spline S156 degree 2 poles (-2.986, -26.5622) (-2.9463, -26.5622) (-2.886, -26.5238) (-2.8634, -26.453) (-2.8634, -26.3671) knots 0 0 0 1 2 3 3 3
  line L165 (-2.8634, -26.3671) -> (-2.8634, -26.2073)
  line L166 (-2.8634, -26.2073) -> (-3.1049, -26.2073)
  dimension "d18" = 0.1
  dimension "d19" = 8
  dimension "d20" = 9
  dimension "d23" = 3.5
  constraints: 2 collinear, 2 end point, 1 midpoint, 1 vertical, 4 other
  measures "d18" distance between parallel lines of L4 L6
  measures "d19" distance between parallel lines of L8 L2
  measures "d20" distance between parallel lines of L3 L5
  measures "d23" distance between parallel lines of L1 L2
emboss "Emboss2" sketch "Sketch4" operation cut depth 0.01 direction (0, 0, -1) draft 1
fillet "Fillet3" radius 0.5 1 edges at (-10.9, 0, 0)
body "Solid1"
